servo_mount_farm (Autodesk Fusion 360 design; units mm, degrees)
Autodesk Fusion 360 part; units mm, degrees
sketch "Sketch1" plane through (0, 0, 0) normal (0, 0, 1) x (1, 0, 0)
  line L0 (-89.8381, 37.0063) -> (-66.5381, 37.0063)
  line L1 (-66.5381, 37.0063) -> (-66.5381, 24.5063)
  line L2 (-66.5381, 24.5063) -> (-89.8381, 24.5063)
  line L3 (-89.8381, 24.5063) -> (-89.8381, 37.0063)
  line L4 (-89.8381, 37.0063) -> (-94.1881, 37.0063)
  line L5 (-94.1881, 37.0063) -> (-94.1881, 24.5063)
  line L6 (-94.1881, 24.5063) -> (-89.8381, 24.5063)
  line L7 (-89.8381, 24.5063) -> (-89.8381, 37.0063)
  line L8 (-66.5381, 37.0063) -> (-62.1881, 37.0063)
  line L9 (-62.1881, 37.0063) -> (-62.1881, 24.5057)
  line L10 (-62.1881, 24.5057) -> (-66.5381, 24.5057)
  line L11 (-66.5381, 24.5057) -> (-66.5381, 37.0063)
  circle A0 centre (-92.1881, 30.7563) radius 1.7
  circle A1 centre (-64.1881, 30.756) radius 1.7
  line L12 (-94.1881, 30.7563) -> (-62.1881, 30.756)
  line L13 (-40.8381, 37.006) -> (-17.5381, 37.006)
  line L14 (-17.5381, 24.4945) -> (-17.5381, 37.006)
  line L15 (-45.1881, 24.506) -> (-40.8381, 24.506)
  circle A2 centre (-43.1881, 30.7557) radius 1.7
  line L16 (-45.1881, 37.006) -> (-45.1881, 24.506)
  line L17 (-17.5381, 37.006) -> (-13.1881, 37.006)
  line L18 (-17.5381, 37.006) -> (-17.5381, 24.506)
  circle A3 centre (-15.1881, 30.7506) radius 1.7
  line L19 (-40.8381, 24.506) -> (-40.8381, 37.006)
  line L20 (-13.1881, 37.006) -> (-13.1881, 24.4945)
  line L21 (-40.8381, 37.006) -> (-45.1881, 37.006)
  line L22 (-17.5381, 24.506) -> (-40.8381, 24.506)
  line L23 (-13.1881, 24.4945) -> (-17.5381, 24.4945)
  line L24 (-45.1881, 30.756) -> (-13.1881, 30.7503)
  line L25 (-40.8381, 24.506) -> (-40.8381, 37.006)
  line L26 (-62.1881, 30.756) -> (-73.1881, 30.756)
  line L27 (-45.1881, 30.756) -> (-34.1881, 30.756)
  line L28 (-94.1881, 141.7563) -> (-62.1881, 141.756)
  line L29 (-94.1881, 135.5063) -> (-89.8381, 135.5063)
  line L30 (-66.5381, 148.0063) -> (-66.5381, 135.5063)
  circle A4 centre (-43.1881, 141.756) radius 1.7
  line L31 (-13.1881, 148.006) -> (-13.1881, 135.506)
  line L32 (-17.5381, 135.506) -> (-40.8381, 135.506)
  line L33 (-45.1881, 141.756) -> (-34.1881, 141.756)
  line L34 (-17.5381, 135.506) -> (-17.5381, 148.006)
  circle A5 centre (-92.1881, 141.7563) radius 1.7
  line L35 (-40.8381, 135.506) -> (-40.8381, 148.006)
  line L36 (-62.1881, 148.0063) -> (-62.1881, 135.5057)
  line L37 (-89.8381, 135.5063) -> (-89.8381, 148.0063)
  line L38 (-17.5381, 148.006) -> (-13.1881, 148.006)
  line L39 (-40.8381, 148.006) -> (-17.5381, 148.006)
  line L40 (-89.8381, 148.0063) -> (-66.5381, 148.0063)
  line L41 (-62.1881, 141.756) -> (-73.1881, 141.756)
  line L42 (-17.5381, 148.006) -> (-17.5381, 135.506)
  line L43 (-66.5381, 148.0063) -> (-62.1881, 148.0063)
  line L44 (-94.1881, 148.0063) -> (-94.1881, 135.5063)
  line L45 (-40.8381, 135.506) -> (-40.8381, 148.006)
  line L46 (-45.1881, 135.506) -> (-40.8381, 135.506)
  line L47 (-13.1881, 135.506) -> (-17.5381, 135.506)
  circle A6 centre (-64.1881, 141.756) radius 1.7
  line L48 (-66.5381, 135.5057) -> (-66.5381, 148.0063)
  line L49 (-40.8381, 148.006) -> (-45.1881, 148.006)
  line L50 (-89.8381, 135.5063) -> (-89.8381, 148.0063)
  line L51 (-66.5381, 135.5063) -> (-89.8381, 135.5063)
  line L52 (-45.1881, 148.006) -> (-45.1881, 135.506)
  line L53 (-62.1881, 135.5057) -> (-66.5381, 135.5057)
  line L54 (-45.1881, 141.756) -> (-13.1881, 141.756)
  line L55 (-89.8381, 148.0063) -> (-94.1881, 148.0063)
  circle A7 centre (-15.1881, 141.756) radius 1.7
  line L56 (-114.1881, 163.0063) -> (6.8119, 163.0063)
  line L57 (6.8119, 163.0063) -> (6.8119, 9.0063)
  line L58 (6.8119, 9.0063) -> (-114.1881, 9.0063)
  line L59 (-114.1881, 9.0063) -> (-114.1881, 163.0063)
  line L60 (195.823, 9.006) -> (74.823, 9.006)
  line L61 (74.823, 163.006) -> (195.823, 163.006)
  line L62 (153.173, 148.006) -> (176.473, 148.006)
  line L63 (195.823, 163.006) -> (195.823, 9.006)
  line L64 (117.473, 135.506) -> (117.473, 148.006)
  line L65 (153.173, 24.506) -> (153.173, 37.006)
  line L66 (176.473, 24.506) -> (153.173, 24.506)
  line L67 (176.473, 30.756) -> (176.473, 24.506)
  line L68 (153.173, 37.006) -> (176.473, 37.006)
  line L69 (153.173, 30.756) -> (159.823, 30.756)
  line L70 (153.173, 24.506) -> (153.173, 37.006)
  line L71 (176.473, 24.506) -> (176.473, 37.006)
  line L72 (153.173, 135.506) -> (153.173, 148.006)
  line L73 (117.473, 135.506) -> (94.173, 135.506)
  line L74 (117.473, 30.756) -> (110.823, 30.756)
  line L75 (94.173, 148.006) -> (117.473, 148.006)
  line L76 (117.473, 148.006) -> (117.473, 135.506)
  line L77 (153.173, 135.506) -> (153.173, 148.006)
  line L78 (117.473, 24.506) -> (117.473, 37.006)
  line L79 (94.173, 135.506) -> (94.173, 148.006)
  line L80 (94.173, 37.006) -> (117.473, 37.006)
  line L81 (94.173, 24.506) -> (94.173, 37.006)
  line L82 (94.173, 135.506) -> (94.173, 148.006)
  line L83 (176.473, 135.506) -> (153.173, 135.506)
  line L84 (176.473, 148.006) -> (176.473, 135.506)
  line L85 (74.823, 9.006) -> (74.823, 163.006)
  line L86 (94.173, 24.506) -> (94.173, 37.006)
  line L87 (117.473, 37.006) -> (117.473, 24.506)
  line L88 (117.473, 24.506) -> (94.173, 24.506)
  line L89 (176.473, 135.506) -> (176.473, 148.006)
  line L90 (87.823, 143.256) -> (182.823, 143.256)
  line L91 (182.823, 143.256) -> (182.823, 29.256)
  line L92 (182.823, 29.256) -> (87.823, 29.256)
  line L93 (87.823, 29.256) -> (87.823, 143.256)
  line L94 (94.173, 30.756) -> (117.473, 30.756)
  line L95 (153.173, 30.756) -> (176.473, 30.756)
  line L96 (94.173, 141.756) -> (117.473, 141.756)
  line L97 (117.473, 141.756) -> (110.823, 141.756)
  line L98 (153.173, 141.756) -> (159.823, 141.756)
  line L99 (153.173, 141.756) -> (176.473, 141.756)
  line L100 (181.073, 105.256) -> (184.573, 105.256)
  line L101 (184.573, 105.256) -> (184.573, 66.756)
  line L102 (184.573, 66.756) -> (181.073, 66.756)
  line L103 (181.073, 66.756) -> (181.073, 105.256)
  line L104 (86.073, 105.256) -> (89.573, 105.256)
  line L105 (89.573, 105.256) -> (89.573, 66.756)
  line L106 (89.573, 66.756) -> (86.073, 66.756)
  line L107 (86.073, 66.756) -> (86.073, 105.256)
  circle A8 centre (-104.1881, 19.0063) radius 1.7
  circle A9 centre (-3.1881, 19.0063) radius 1.7
  circle A10 centre (-104.1881, 153.0063) radius 1.7
  circle A11 centre (-3.1881, 153.0063) radius 1.7
  line L108 (-62.1881, 30.756) -> (-45.1881, 30.756)
  line L109 (-62.1881, 141.756) -> (-45.1881, 141.756)
  line L110 (-53.6881, 30.756) -> (-53.6881, 141.756)
  point P0 (-78.1881, 30.7562)
  point P1 (-29.1881, 30.7531)
  point P2 (-78.1881, 141.7562)
  point P3 (-29.1881, 141.756)
  point P4 (105.823, 30.756)
  point P5 (105.823, 141.756)
  point P6 (164.823, 141.756)
  point P7 (164.823, 30.756)
  dimension "d1" = 23.3
  dimension "d2" = 12.5
  dimension "d6" = 12.5
  dimension "d7" = 32
  dimension "d8" = 3.4
  dimension "d9" = 3.4
  dimension "d10" = 28
  dimension "d13" = 14
  dimension "d14" = 23.3
  dimension "d15" = 12.5
  dimension "d16" = 12.5
  dimension "d17" = 32
  dimension "d18" = 3.4
  dimension "d19" = 3.4
  dimension "d20" = 28
  dimension "d21" = 14
  dimension "d22" = 11
  dimension "d23" = 11
  dimension "d24" = 39
  dimension "d25" = 23.3
  dimension "d26" = 12.5
  dimension "d27" = 12.5
  dimension "d28" = 32
  dimension "d29" = 3.4
  dimension "d30" = 3.4
  dimension "d31" = 28
  dimension "d32" = 14
  dimension "d33" = 23.3
  dimension "d34" = 12.5
  dimension "d35" = 12.5
  dimension "d36" = 32
  dimension "d37" = 3.4
  dimension "d38" = 3.4
  dimension "d39" = 28
  dimension "d40" = 14
  dimension "d41" = 11
  dimension "d42" = 11
  dimension "d43" = 39
  dimension "d44" = 121
  dimension "d45" = 154
  dimension "d46" = 111
  dimension "d47" = 15
  dimension "d48" = 20
  dimension "d51" = 23.3
  dimension "d52" = 12.5
  dimension "d53" = 12.5
  dimension "d59" = 23.3
  dimension "d60" = 12.5
  dimension "d61" = 12.5
  dimension "d69" = 49
  dimension "d70" = 23.3
  dimension "d71" = 12.5
  dimension "d72" = 12.5
  dimension "d78" = 23.3
  dimension "d79" = 12.5
  dimension "d80" = 12.5
  dimension "d88" = 49
  dimension "d89" = 121
  dimension "d90" = 154
  dimension "d92" = 15
  dimension "d94" = 95
  dimension "d95" = 114
  dimension "d96" = 1.5
  dimension "d97" = 13
  dimension "d98" = 3.5
  dimension "d99" = 38.5
  dimension "d100" = 37.5
  dimension "d101" = 1.75
  dimension "d102" = 3.5
  dimension "d103" = 38.5
  dimension "d104" = 1.75
  dimension "d105" = 37.5
  dimension "d117" = 3.4
  dimension "d118" = 10
  dimension "d119" = 10
  dimension "d122" = 101
  dimension "d123" = 134
  constraint horizontal L0
  constraint vertical L1
  constraint horizontal L2
  constraint vertical L3
  constraint horizontal L4
  constraint vertical L5
  constraint horizontal L6
  constraint vertical L7
  constraint horizontal L8
  constraint vertical L9
  constraint horizontal L10
  constraint vertical L11
  constraint equal L4 L8
  constraint midpoint L5 L12.start
  constraint midpoint L9 L12.end
  constraint coincident A0.centre L12
  constraint coincident A1.centre L12
  constraint midpoint P0 L12
  constraint horizontal L13
  constraint vertical L18
  constraint horizontal L22
  constraint vertical L25
  constraint horizontal L21
  constraint vertical L16
  constraint horizontal L15
  constraint vertical L19
  constraint horizontal L17
  constraint vertical L20
  constraint horizontal L23
  constraint vertical L14
  constraint equal L17 L21
  constraint midpoint L24.start L16
  constraint midpoint L24.end L20
  constraint coincident A2.centre L24
  constraint coincident A3.centre L24
  constraint midpoint P1 L24
  constraint perpendicular L9 L26
  constraint perpendicular L16 L27
  constraint horizontal L40
  constraint vertical L30
  constraint horizontal L51
  constraint vertical L37
  constraint horizontal L55
  constraint vertical L44
  constraint horizontal L29
  constraint vertical L50
  constraint horizontal L43
  constraint vertical L36
  constraint horizontal L53
  constraint vertical L48
  constraint equal L43 L55
  constraint midpoint L28.start L44
  constraint midpoint L28.end L36
  constraint coincident A5.centre L28
  constraint coincident A6.centre L28
  constraint midpoint P2 L28
  constraint horizontal L39
  constraint vertical L42
  constraint horizontal L32
  constraint vertical L35
  constraint horizontal L49
  constraint vertical L52
  constraint horizontal L46
  constraint vertical L45
  constraint horizontal L38
  constraint vertical L31
  constraint horizontal L47
  constraint vertical L34
  constraint equal L38 L49
  constraint midpoint L33.start L52
  constraint midpoint L54.end L31
  constraint coincident A4.centre L54
  constraint coincident A7.centre L54
  constraint midpoint P3 L54
  constraint perpendicular L36 L41
  constraint perpendicular L33 L52
  constraint horizontal L56
  constraint vertical L57
  constraint horizontal L58
  constraint vertical L59
  constraint horizontal L80
  constraint vertical L87
  constraint horizontal L88
  constraint vertical L81
  constraint vertical L86
  constraint vertical L78
  constraint horizontal L68
  constraint vertical L67
  constraint horizontal L66
  constraint vertical L70
  constraint vertical L65
  constraint vertical L71
  constraint horizontal L75
  constraint vertical L76
  constraint horizontal L73
  constraint vertical L82
  constraint vertical L79
  constraint vertical L64
  constraint horizontal L62
  constraint vertical L84
  constraint horizontal L83
  constraint vertical L72
  constraint vertical L77
  constraint vertical L89
  constraint horizontal L61
  constraint vertical L63
  constraint horizontal L60
  constraint vertical L85
  constraint horizontal L90
  constraint vertical L91
  constraint horizontal L92
  constraint vertical L93
  constraint coincident L78 L74.start
  constraint coincident L65 L69.start
  constraint coincident L81 L94.start
  constraint coincident L64 L96.end
  constraint coincident L84 L99.end
  constraint coincident L72 L98.start
  constraint coincident L79 L96.start
  constraint horizontal L100
  constraint vertical L101
  constraint horizontal L102
  constraint vertical L103
  constraint horizontal L104
  constraint vertical L105
  constraint horizontal L106
  constraint vertical L107
  constraint perpendicular L16 L108
  constraint parallel L33 L109
  constraint midpoint L108 L110.start
  constraint midpoint L109 L110.end
  constraint perpendicular L109 L110
  measures "d1" distance of L0.start L0.end
  measures "d2" distance of L0.start L2.end
  measures "d6" distance of L0.start L2.end
  measures "d7" distance of L4.end L8.end
  measures "d8" diameter of A0
  measures "d9" diameter of A1
  measures "d10" distance of A0.centre A1.centre
  measures "d13" distance of A1.centre P0
  measures "d14" distance of L13.end L13.start
  measures "d15" distance of L13.start L15.end
  measures "d16" distance of L15.end L13.start
  measures "d17" distance of L16.start L17.end
  measures "d18" diameter of A2
  measures "d19" diameter of A3
  measures "d20" distance of A3.centre A2.centre
  measures "d21" distance of A3.centre P1
  measures "d22" distance of L12.end L26.end
  measures "d23" distance of L24.start L27.end
  measures "d24" distance of L26.end L27.end
  measures "d25" distance of L30.start L37.end
  measures "d26" distance of L37.end L29.end
  measures "d27" distance of L29.end L37.end
  measures "d28" distance of L44.start L36.start
  measures "d29" diameter of A5
  measures "d30" diameter of A6
  measures "d31" distance of A6.centre A5.centre
  measures "d32" distance of A6.centre P2
  measures "d33" distance of L34.end L35.end
  measures "d34" distance of L32.end L35.end
  measures "d35" distance of L32.end L35.end
  measures "d36" distance of L49.end L31.start
  measures "d37" diameter of A4
  measures "d38" diameter of A7
  measures "d39" distance of A4.centre A7.centre
  measures "d40" distance of P3 A7.centre
  measures "d41" distance of L28.end L41.end
  measures "d42" distance of L33.end L33.start
  measures "d43" distance of L33.end L41.end
  measures "d44" distance of L56.start L56.end
  measures "d45" distance of L56.start L58.end
  measures "d46" distance of L12 L28
  measures "d47" distance of L40 L56
  measures "d48" distance of L5 L59
  measures "d51" distance of L78.end L80.start
  measures "d52" distance of L80.start L81.start
  measures "d53" distance of L81.start L80.start
  measures "d59" distance of L68.end L65.end
  measures "d60" distance of L65.start L65.end
  measures "d61" distance of L65.start L65.end
  measures "d69" distance of L69.end L74.end
  measures "d70" distance of L64.end L75.start
  measures "d71" distance of L75.start L73.end
  measures "d72" distance of L73.end L75.start
  measures "d78" distance of L62.end L62.start
  measures "d79" distance of L62.start L72.start
  measures "d80" distance of L72.start L62.start
  measures "d88" distance of L98.end L97.end
  measures "d89" distance of L61.start L61.end
  measures "d90" distance of L61.start L60.end
  measures "d92" distance of L61 L75
  measures "d94" distance of L90.start L90.end
  measures "d95" distance of L90.start L92.end
  measures "d96" distance of L90 L99
  measures "d97" distance of L63 L91
  measures "d98" distance of L100.start L100.end
  measures "d99" distance of L100.start L102.end
  measures "d100" distance of L91.end L102
  measures "d101" distance of L91 L101
  measures "d102" distance of L104.start L104.end
  measures "d103" distance of L104.start L106.end
  measures "d104" distance of L93 L107
  measures "d105" distance of L92 L106
  measures "d117" diameter of A8
  measures "d118" distance of L58 A8.centre
  measures "d119" distance of L59 A8.centre
extrude "Extrude1" add sketch "Sketch1" along normal blind 2 contours L3 L4 L5 L7 A0 L12 | L1 L8 L9 L11 A1 L12 L26 | L3 L5 L6 L7 A0 L12 | L1 L9 L10 L11 A1 L12 L26 | A2 L16 L19 L21 L24 L25 L27 | L14 L17 L18 A3 L20 L24 | L15 A2 L16 L19 L24 L25 L27 | L14 L18 A3 L20 L23 L24 | L28 L30 L36 L41 L43 A6 L48 | L28 L30 L36 L41 A6 L48 L53 | L28 A5 L37 L44 L50 L55 | L28 L29 A5 L37 L44 L50 | A4 L33 L35 L45 L46 L52 L54 | A4 L33 L35 L45 L49 L52 L54 | L31 L34 L42 L47 L54 A7 | L31 L34 L38 L42 L54 A7 | L56 L57 L58 L59 makes body 1
extrude "Extrude2" add sketch "Sketch1" along normal blind 2 separate body contours L60 L61 L63 L85 | L64 L65 L67 L68 L70 L71 L72 L73 L76 L77 L78 L79 L80 L81 L82 L83 L84 L86 L87 L89 L90 L91 L92 L93 L100 L102 L103 L104 L105 L106 makes body 2
sketch "Sketch2" plane through (0, 0, 2) normal (0, 0, 1) x (-1, 0, 0)
  line L0 (-176.473, -135.506) -> (-153.173, -135.506)
  line L1 (-153.173, -135.506) -> (-153.173, -148.006)
  line L2 (-153.173, -148.006) -> (-176.473, -148.006)
  line L3 (-176.473, -148.006) -> (-176.473, -135.506)
  line L4 (-184.573, -66.756) -> (-181.073, -66.756)
  line L5 (-181.073, -66.756) -> (-181.073, -105.256)
  line L6 (-181.073, -105.256) -> (-184.573, -105.256)
  line L7 (-184.573, -105.256) -> (-184.573, -66.756)
  line L8 (-89.573, -66.756) -> (-86.073, -66.756)
  line L9 (-86.073, -66.756) -> (-86.073, -105.256)
  line L10 (-86.073, -105.256) -> (-89.573, -105.256)
  line L11 (-89.573, -105.256) -> (-89.573, -66.756)
  line L12 (-117.473, -135.506) -> (-94.173, -135.506)
  line L13 (-94.173, -135.506) -> (-94.173, -148.006)
  line L14 (-94.173, -148.006) -> (-117.473, -148.006)
  line L15 (-117.473, -148.006) -> (-117.473, -135.506)
  line L16 (-176.473, -24.506) -> (-153.173, -24.506)
  line L17 (-153.173, -24.506) -> (-153.173, -37.006)
  line L18 (-153.173, -37.006) -> (-176.473, -37.006)
  line L19 (-176.473, -37.006) -> (-176.473, -24.506)
  line L20 (-117.473, -37.006) -> (-117.473, -24.506)
  line L21 (-117.473, -24.506) -> (-94.173, -24.506)
  line L22 (-94.173, -24.506) -> (-94.173, -37.006)
  line L23 (-94.173, -37.006) -> (-117.473, -37.006)
  line L24 (-74.823, -9.006) -> (-195.823, -9.006)
  line L25 (-195.823, -9.006) -> (-195.823, -163.006)
  line L26 (-195.823, -163.006) -> (-74.823, -163.006)
  line L27 (-74.823, -163.006) -> (-74.823, -9.006)
  line L28 (-94.173, -148.006) -> (-176.473, -148.006)
  line L29 (-176.473, -148.006) -> (-176.473, -135.506)
  line L30 (-176.473, -135.506) -> (-94.173, -135.506)
  line L31 (-94.173, -135.506) -> (-94.173, -148.006)
  line L32 (-94.173, -37.006) -> (-176.473, -37.006)
  line L33 (-176.473, -37.006) -> (-176.473, -24.506)
  line L34 (-176.473, -24.506) -> (-94.173, -24.506)
  line L35 (-94.173, -24.506) -> (-94.173, -37.006)
  line L36 (-130.323, -135.506) -> (-140.323, -135.506)
  line L37 (-140.323, -135.506) -> (-140.323, -37.006)
  line L38 (-140.323, -37.006) -> (-130.323, -37.006)
  line L39 (-130.323, -37.006) -> (-130.323, -135.506)
  circle A0 centre (-84.823, -153.006) radius 1.7
  circle A1 centre (-185.823, -153.006) radius 1.7
  circle A2 centre (-84.823, -19.006) radius 1.7
  circle A3 centre (-185.823, -19.006) radius 1.7
  line L40 (-94.173, -148.006) -> (-84.173, -148.006)
  line L41 (-84.173, -148.006) -> (-84.173, -135.506)
  line L42 (-84.173, -135.506) -> (-94.173, -135.506)
  line L43 (-94.173, -135.506) -> (-94.173, -148.006)
  line L44 (-176.473, -148.006) -> (-186.473, -148.006)
  line L45 (-186.473, -148.006) -> (-186.473, -135.506)
  line L46 (-186.473, -135.506) -> (-176.473, -135.506)
  line L47 (-176.473, -135.506) -> (-176.473, -148.006)
  line L48 (-94.173, -37.006) -> (-84.173, -37.006)
  line L49 (-84.173, -37.006) -> (-84.173, -24.506)
  line L50 (-84.173, -24.506) -> (-94.173, -24.506)
  line L51 (-94.173, -24.506) -> (-94.173, -37.006)
  line L52 (-176.473, -24.506) -> (-186.473, -24.506)
  line L53 (-186.473, -24.506) -> (-186.473, -37.006)
  line L54 (-186.473, -37.006) -> (-176.473, -37.006)
  line L55 (-176.473, -37.006) -> (-176.473, -24.506)
  point P0 (-185.823, -153.006)
  point P1 (-84.823, -19.006)
  point P2 (-185.823, -19.006)
  point P3 (-185.823, -153.006)
  point P4 (-84.823, -19.006)
  point P5 (-185.823, -19.006)
  dimension "d108" = 10
  dimension "d109" = 36.15
  dimension "d110" = 3.4
  dimension "d111" = 10
  dimension "d112" = 10
  dimension "d115" = -101
  dimension "d116" = 134
  dimension "d126" = -101
  dimension "d127" = 134
  dimension "d130" = -101
  dimension "d131" = 134
  dimension "d137" = 10
  dimension "d138" = 12.5
  dimension "d139" = 10
  dimension "d140" = 12.5
  dimension "d141" = 10
  dimension "d142" = 12.5
  dimension "d143" = 10
  dimension "d144" = 12.5
  constraint horizontal L28
  constraint vertical L29
  constraint horizontal L30
  constraint vertical L31
  constraint coincident L0.start L3.end
  constraint coincident L13.end L14.start
  constraint horizontal L32
  constraint vertical L33
  constraint horizontal L34
  constraint vertical L35
  constraint coincident L16.start L19.end
  constraint coincident L22.end L23.start
  constraint horizontal L36
  constraint vertical L37
  constraint horizontal L38
  constraint vertical L39
  constraint coincident L32 L37.end
  constraint coincident L30 L36.start
  constraint horizontal L40
  constraint vertical L41
  constraint horizontal L42
  constraint vertical L43
  constraint horizontal L44
  constraint vertical L45
  constraint horizontal L46
  constraint vertical L47
  constraint coincident L2.end L3.start
  constraint horizontal L48
  constraint vertical L49
  constraint horizontal L50
  constraint vertical L51
  constraint horizontal L52
  constraint vertical L53
  constraint horizontal L54
  constraint vertical L55
  measures "d108" distance of L37 L39
  measures "d109" distance of L12.end L39
  measures "d110" diameter of A0
  measures "d111" distance of L26 A0.centre
  measures "d112" distance of L27 A0.centre
  measures "d137" distance of L13.end L40.end
  measures "d138" distance of L13.end L12.end
  measures "d139" distance of L2.end L44.end
  measures "d140" distance of L2.end L0.start
  measures "d141" distance of L22.end L48.end
  measures "d142" distance of L22.end L21.end
  measures "d143" distance of L16.start L52.end
  measures "d144" distance of L16.start L18.end
extrude "Extrude3" cut sketch "Sketch2" against normal through all contours A0 bodies 2
extrude "Extrude4" cut sketch "Sketch2" against normal through all contours A3 bodies 2
extrude "Extrude5" cut sketch "Sketch2" against normal through all contours A1 bodies 2
extrude "Extrude6" cut sketch "Sketch2" against normal through all contours A2 bodies 2
extrude "Extrude7" cut sketch "Sketch2" against normal through all contours L3 L29 L44 L45 L46 L47 | L1 L15 L28 L30 L36 | L30 L32 L36 L37 L38 L39 | L17 L20 L32 L34 L38 | L13 L31 L40 L41 L42 L43 | L19 L33 L52 L53 L54 L55 | L22 L35 L48 L49 L50 L51 bodies 2
sketch "Sketch4" plane through (0, 0, 2) normal (0, 0, 1) x (-1, 0, 0)
  circle A0 centre (64.1881, -30.756) radius 1.7
  circle A1 centre (43.1881, -141.756) radius 1.7
  line L0 (66.5381, -24.5063) -> (89.8381, -24.5063)
  line L1 (89.8381, -24.5063) -> (89.8381, -37.0063)
  line L2 (89.8381, -37.0063) -> (66.5381, -37.0063)
  line L3 (66.5381, -37.0063) -> (66.5381, -24.5063)
  circle A2 centre (3.1881, -19.0063) radius 1.7
  circle A3 centre (15.1881, -141.756) radius 1.7
  circle A4 centre (15.1881, -30.7506) radius 1.7
  circle A5 centre (104.1881, -19.0063) radius 1.7
  circle A6 centre (64.1881, -141.756) radius 1.7
  circle A7 centre (3.1881, -153.0063) radius 1.7
  line L4 (17.5381, -24.506) -> (40.8381, -24.506)
  line L5 (40.8381, -24.506) -> (40.8381, -37.006)
  line L6 (40.8381, -37.006) -> (17.5381, -37.006)
  line L7 (17.5381, -37.006) -> (17.5381, -24.506)
  circle A8 centre (43.1881, -30.7557) radius 1.7
  circle A9 centre (92.1881, -141.7563) radius 1.7
  line L8 (66.5381, -148.0063) -> (66.5381, -135.5063)
  line L9 (66.5381, -135.5063) -> (89.8381, -135.5063)
  line L10 (89.8381, -135.5063) -> (89.8381, -148.0063)
  line L11 (89.8381, -148.0063) -> (66.5381, -148.0063)
  circle A10 centre (92.1881, -30.7563) radius 1.7
  circle A11 centre (104.1881, -153.0063) radius 1.7
  line L12 (17.5381, -135.506) -> (40.8381, -135.506)
  line L13 (40.8381, -135.506) -> (40.8381, -148.006)
  line L14 (40.8381, -148.006) -> (17.5381, -148.006)
  line L15 (17.5381, -148.006) -> (17.5381, -135.506)
  line L16 (114.1881, -9.0063) -> (-6.8119, -9.0063)
  line L17 (-6.8119, -9.0063) -> (-6.8119, -163.0063)
  line L18 (-6.8119, -163.0063) -> (114.1881, -163.0063)
  line L19 (114.1881, -163.0063) -> (114.1881, -9.0063)
  line L20 (-74.823, -9.006) -> (-195.823, -9.006)
  line L21 (-195.823, -9.006) -> (-195.823, -163.006)
  line L22 (-195.823, -163.006) -> (-74.823, -163.006)
  line L23 (-74.823, -163.006) -> (-74.823, -9.006)
  line L24 (-89.573, -66.756) -> (-86.073, -66.756)
  line L25 (-86.073, -66.756) -> (-86.073, -105.256)
  line L26 (-86.073, -105.256) -> (-89.573, -105.256)
  line L27 (-89.573, -105.256) -> (-89.573, -66.756)
  line L28 (-184.573, -66.756) -> (-181.073, -66.756)
  line L29 (-181.073, -66.756) -> (-181.073, -105.256)
  line L30 (-181.073, -105.256) -> (-184.573, -105.256)
  line L31 (-184.573, -105.256) -> (-184.573, -66.756)
  circle A12 centre (-84.823, -153.006) radius 1.7
  circle A13 centre (-185.823, -19.006) radius 1.7
  circle A14 centre (-185.823, -153.006) radius 1.7
  circle A15 centre (-84.823, -19.006) radius 1.7
  line L32 (-84.173, -37.006) -> (-130.323, -37.006)
  line L33 (-130.323, -37.006) -> (-130.323, -135.506)
  line L34 (-130.323, -135.506) -> (-84.173, -135.506)
  line L35 (-84.173, -148.006) -> (-186.473, -148.006)
  line L36 (-186.473, -135.506) -> (-140.323, -135.506)
  line L37 (-140.323, -135.506) -> (-140.323, -37.006)
  line L38 (-140.323, -37.006) -> (-186.473, -37.006)
  line L39 (-186.473, -24.506) -> (-84.173, -24.506)
  line L40 (-84.173, -135.506) -> (-84.173, -148.006)
  line L41 (-186.473, -148.006) -> (-186.473, -135.506)
  line L42 (-186.473, -37.006) -> (-186.473, -24.506)
  line L43 (-84.173, -24.506) -> (-84.173, -37.006)
